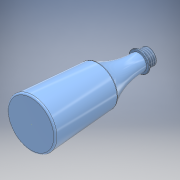
# Autodesk Inventor part: flaska
Saved by Autodesk Inventor 2018 (Build 220112000, 112)
## iProperties
Created: 2018-06-14
Part Number: flaska
Material: Generic
Document SubType Name: Modeling
Designer: dilan haddad
Density: 1 g/cm^3
Appearance: Default
Author: dilan haddad
Autodesk Inventor part; units mm, degrees
ref_plane "YZ Plane" through (0, 0, 0) normal (1, 0, 0) x (0, 1, 0)
ref_plane "XZ Plane" through (0, 0, 0) normal (0, 1, 0) x (-1, 0, 0)
ref_plane "XY Plane" through (0, 0, 0) normal (0, 0, 1) x (1, 0, 0)
sketch "Sketch1" plane through (0, 0, 0) normal (0, 0, 1) x (1, 0, 0)
  line L0 (0, 0) -> (0, 150)
  line L1 (0, 0) -> (31, 0)
  line L2 (0, 150) -> (10, 150)
  line L3 (10, 150) -> (10, 139)
  line L4 (10, 139) -> (13, 139)
  line L5 (13, 139) -> (13, 137)
  line L6 (13, 137) -> (10, 137)
  arc A0 (10, 137) -> (25, 85) centre (104.4877, 136.0926) ccw
  line L7 (25, 85) -> (31, 0)
  constraints: 16 end point, 4 perpendicular, 2 horizontal, 2 point on circle, 1 centre point, 1 point on line
revolve "Revolution1" add sketch "Sketch1" angle 360 about axis through (0, 0, 0) along (0, 1, 0)
shell "Shell1" thickness 1 removed faces 1 at (-1.6385, 150, 0.6428)
fillet "Fillet1" radius 2 1 edges at (-25, 85, 0)
fillet "Fillet2" radius 2 1 edges at (-31, 0, 0)
fillet "Fillet3" radius 0.5 4 edges at (-10, 150, 0) (-9, 150, 0) (-13, 139, 0) (-13, 137, 0)
thread "Thread1" size "M20x2.5" class "6g" standard "ANSI Metric M Profile" full length
sketch "Sketch2" plane through (0, 139, 0) normal (0, 1, 0) x (1, 0, 0)
  point P0 (0, 0)
sketch "Sketch3" plane through (0, 1, 0) normal (0, 1, 0) x (1, 0, 0)
  point P0 (0, 0)
body "Solid1"
